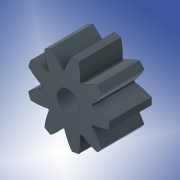
# Autodesk Inventor part: GA002
Saved by Autodesk Inventor 2017 SP1 (Build 210196100, 196)
## iProperties
Created: 2017-06-20
Part Number: GA002
Material: ABS Plastic
Document SubType Name: Modeling
Designer: zallen
Density: 1.06 g/cm^3
Appearance: CR Dark Blue
Author: zallen
Autodesk Inventor part; units mm, degrees
ref_plane "YZ Plane" through (0, 0, 0) normal (1, 0, 0) x (0, 1, 0)
ref_plane "XZ Plane" through (0, 0, 0) normal (0, 1, 0) x (-1, 0, 0)
ref_plane "XY Plane" through (0, 0, 0) normal (0, 0, 1) x (1, 0, 0)
sketch "Sketch1" plane through (0, 0, 0) normal (0, 0, 1) x (1, 0, 0)
  circle A0 centre (0, 0) radius 6
  circle A1 centre (0, 0) radius 2.6
  dimension "d0" = 12
  dimension "d1" = 5.2
  constraints: 2 centre point, 2 coincident
  measures "d0" diameter of A0
  measures "d1" diameter of A1
extrude "Extrusion1" add sketch "Sketch1" along normal blind 10
sketch "Sketch3" plane through (0, 0, 10) normal (0, 0, 1) x (1, 0, 0)
  line L0 (0, 0) -> (25, 0) construction
  arc A0 (9.6912, 0.8) -> (5.6912, 1.9) centre (3.7521, -12.9741) ccw
  circle A1 centre (0, 0) radius 6 projected
  arc A2 (9.6912, -0.8) -> (9.6912, 0.8) centre (-10.2928, 0) ccw
  arc A3 (5.6912, -1.9) -> (9.6912, -0.8) centre (3.7521, 12.9741) ccw
  arc A4 (5.6912, -1.9) -> (5.6912, 1.9) centre (0, 0) ccw
  arc A5 (6.9097, 6.8422) -> (3.1384, 5.1137) centre (11.2139, -7.527) ccw
  arc A6 (7.9381, 5.6166) -> (6.9097, 6.8422) centre (-7.8847, -6.6161) ccw
  arc A7 (5.581, 2.2028) -> (7.9381, 5.6166) centre (-5.4653, 12.3506) ccw
  arc A8 (5.581, 2.2028) -> (3.1384, 5.1137) centre (0, 0) ccw
  arc A9 (0.895, 9.6829) -> (-0.8829, 5.9347) centre (13.4286, 1.4421) ccw
  arc A10 (2.4707, 9.4051) -> (0.895, 9.6829) centre (-1.7873, -10.1364) ccw
  arc A11 (2.8594, 5.2748) -> (2.4707, 9.4051) centre (-12.1255, 5.948) ccw
  arc A12 (2.8594, 5.2748) -> (-0.8829, 5.9347) centre (0, 0) ccw
  arc A13 (-5.5384, 7.9928) -> (-4.4911, 3.9787) centre (9.3599, 9.7365) ccw
  arc A14 (-4.1528, 8.7928) -> (-5.5384, 7.9928) centre (5.1464, -8.9138) ccw
  arc A15 (-1.2002, 5.8787) -> (-4.1528, 8.7928) centre (-13.112, -3.2377) ccw
  arc A16 (-1.2002, 5.8787) -> (-4.4911, 3.9787) centre (0, 0) ccw
  arc A17 (-9.3804, 2.5628) -> (-5.9978, 0.1611) centre (0.9116, 13.475) ccw
  arc A18 (-8.8332, 4.0663) -> (-9.3804, 2.5628) centre (9.672, -3.5203) ccw
  arc A19 (-4.6982, 3.7319) -> (-8.8332, 4.0663) centre (-7.9632, -10.9084) ccw
  arc A20 (-4.6982, 3.7319) -> (-5.9978, 0.1611) centre (0, 0) ccw
  arc A21 (-8.8332, -4.0663) -> (-4.6982, -3.7319) centre (-7.9632, 10.9084) ccw
  arc A22 (-9.3804, -2.5628) -> (-8.8332, -4.0663) centre (9.672, 3.5203) ccw
  arc A23 (-5.9978, -0.1611) -> (-9.3804, -2.5628) centre (0.9116, -13.475) ccw
  arc A24 (-5.9978, -0.1611) -> (-4.6982, -3.7319) centre (0, 0) ccw
  arc A25 (-4.1528, -8.7928) -> (-1.2002, -5.8787) centre (-13.112, 3.2377) ccw
  arc A26 (-5.5384, -7.9928) -> (-4.1528, -8.7928) centre (5.1464, 8.9138) ccw
  arc A27 (-4.4911, -3.9787) -> (-5.5384, -7.9928) centre (9.3599, -9.7365) ccw
  arc A28 (-4.4911, -3.9787) -> (-1.2002, -5.8787) centre (0, 0) ccw
  arc A29 (2.4707, -9.4051) -> (2.8594, -5.2748) centre (-12.1255, -5.948) ccw
  arc A30 (0.895, -9.6829) -> (2.4707, -9.4051) centre (-1.7873, 10.1364) ccw
  arc A31 (-0.8829, -5.9347) -> (0.895, -9.6829) centre (13.4286, -1.4421) ccw
  arc A32 (-0.8829, -5.9347) -> (2.8594, -5.2748) centre (0, 0) ccw
  arc A33 (7.9381, -5.6166) -> (5.581, -2.2028) centre (-5.4653, -12.3506) ccw
  arc A34 (6.9097, -6.8422) -> (7.9381, -5.6166) centre (-7.8847, 6.6161) ccw
  arc A35 (3.1384, -5.1137) -> (6.9097, -6.8422) centre (11.2139, 7.527) ccw
  arc A36 (3.1384, -5.1137) -> (5.581, -2.2028) centre (0, 0) ccw
  point P0 (9.7072, 0)
  point P1 (7.4362, 6.2397)
  point P2 (1.6856, 9.5598)
  point P3 (-4.8536, 8.4067)
  point P4 (-9.1218, 3.3201)
  point P5 (-9.1218, -3.3201)
  point P6 (-4.8536, -8.4067)
  point P7 (1.6856, -9.5598)
  point P8 (7.4362, -6.2397)
  dimension "d8" = 25
  dimension "d9" = 15
  dimension "d10" = 1.6
  dimension "d11" = 20
  dimension "d12" = 4
  dimension "d13" = 1.1
  dimension "d14" = 15
  dimension "d15" = 1.1
  dimension "d16" = 4
  dimension "d19" = 360
  constraints: 75 point on circle, 36 centre point, 2 end point, 1 concentric, 1 horizontal, 1 point on line, 118 other
  measures "d8" distance of L0.start L0.end
  measures "d9" radius of A0
  measures "d10" distance of A0.start A2.start
  measures "d11" radius of A2
  measures "d12" horizontal distance of A0.start A0.end
  measures "d13" vertical distance of A0.start A0.end
  measures "d14" radius of A3
  measures "d15" vertical distance of A2.start A1.end
  measures "d16" horizontal distance of A1.end A2.start
extrude "Extrusion3" add sketch "Sketch3" against normal blind 10 contours A2 A3 A1 A0 | A1 A5 A6 A7 | A33 A34 A35 A1 | A1 A9 A10 A11 | A29 A30 A31 A1 | A1 A13 A14 A15 | A25 A26 A27 A1 | A1 A17 A18 A19 | A21 A22 A23 A1
body "Solid1"
